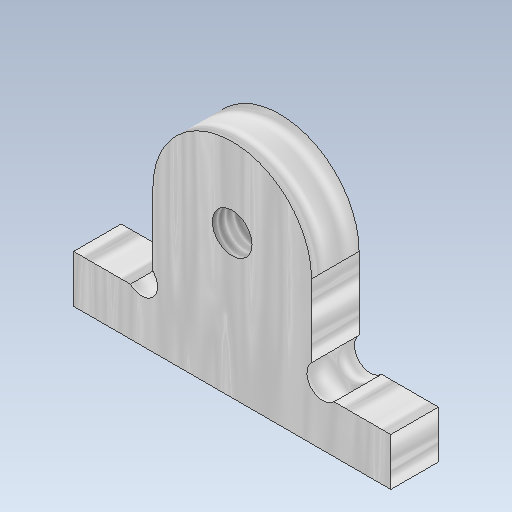
# Autodesk Inventor part: T字金具M3
Saved by Autodesk Inventor 2020.2 (Build 242310000, 310)
## iProperties
Created: 2020-03-23
Part Number: T字金具M3
Material: アルミニウム 7075
Document SubType Name: Modeling
Designer: aoyam
Density: 2.81 g/cm^3
Appearance: サテン - ブラシ仕上げ 重厚
Author: aoyam
Autodesk Inventor part; units mm, degrees
ref_plane "YZ Plane" through (0, 0, 0) normal (1, 0, 0) x (0, 1, 0)
ref_plane "XZ Plane" through (0, 0, 0) normal (0, 1, 0) x (-1, 0, 0)
ref_plane "XY Plane" through (0, 0, 0) normal (0, 0, 1) x (1, 0, 0)
sketch "スケッチ1" plane through (0, 0, 0) normal (0, 0, 1) x (1, 0, 0)
  circle A0 centre (0, 0) radius 1.25
  circle A1 centre (0, 0) radius 5
  line L0 (-10, -6) -> (10, -6)
  line L1 (10, -6) -> (10, -9)
  line L2 (10, -9) -> (-10, -9)
  line L3 (-10, -9) -> (-10, -6)
  line L4 (-5, 0) -> (-5, -6)
  line L5 (5, 0) -> (5, -6)
  circle A2 centre (-5.7106, -5.2894) radius 1.005
  circle A3 centre (5.7106, -5.2894) radius 1.005
  line L6 (-5.7106, -5.2894) -> (-5, -6)
  line L7 (5.7106, -5.2894) -> (5, -6)
  point P0 (6.4213, -6)
  point P1 (5, -4.5787)
  point P2 (-5, -4.5787)
  point P3 (-6.4213, -6)
  dimension "d7" = 2.01
  dimension "d8" = 2.01
  dimension "d0" = 2.5
  dimension "d1" = 10
  dimension "d2" = 3
  dimension "d3" = 20
  dimension "d4" = 6
  dimension "d5" = 5
  dimension "d6" = 6
  dimension "d9" = 45
  dimension "d10" = 45
  constraints: 16 end point, 5 perpendicular, 3 coincident, 2 centre point, 2 point on circle, 2 point on line, 1 horizontal, 1 tangent, 6 other
  measures "d0" diameter of A0
  measures "d1" diameter of A1
  measures "d2" distance of L0.end L1.end
  measures "d3" distance of L1.end L2.end
  measures "d4" distance from line of L0 A1.centre
  measures "d5" distance of L0.end L5.end
  measures "d6" distance of L4.start L4.end
  measures "d9" angle of L4 L6
  measures "d10" angle of L5 L7
extrude "押し出し1" add sketch "スケッチ1" along normal blind 3 contours A1 | L5 A3 L0 A2 L4 A1 | A3 L0 L1 L2 L3 A2
thread "ねじ1" size "M3x0.5" class "6H" standard "ANSI Metric M Profile" full length
sketch "スケッチ2" plane through (0, 0, 3) normal (0, 0, 1) x (1, 0, 0)
  line L0 (-10, -6) -> (-10, -9) projected
  line L1 (-10, -9) -> (10, -9) projected
  line L2 (10, -9) -> (10, -6) projected
  line L3 (10, -6) -> (6.4213, -6) projected
  arc A0 (5, -4.5787) -> (6.4213, -6) centre (5.7106, -5.2894) ccw projected
  line L4 (5, -4.5787) -> (5, 0) projected
  arc A1 (5, 0) -> (-5, 0) centre (0, 0) ccw projected
  line L5 (-5, 0) -> (-5, -4.5787) projected
  arc A2 (-6.4213, -6) -> (-5, -4.5787) centre (-5.7106, -5.2894) ccw projected
  line L6 (-6.4213, -6) -> (-10, -6) projected
  circle A3 centre (0, 0) radius 1.25 projected
